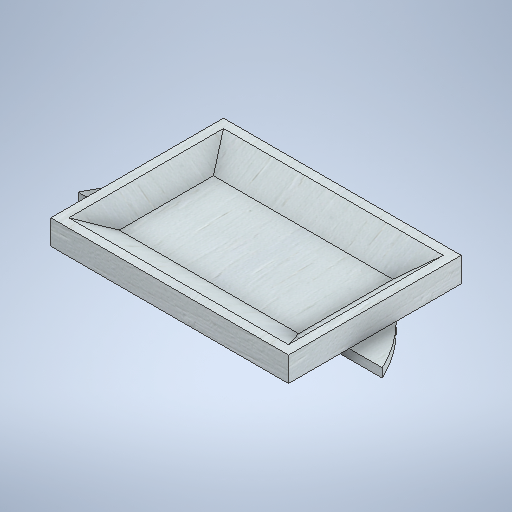
# Autodesk Inventor part: Soporte_caja
Saved by Autodesk Inventor 2025.2 (Build 292293000, 293)
## iProperties
Created: 2025-11-06
Part Number: Soporte_caja
Material: Genérico
Document SubType Name: Modeling
Designer: Dax
Density: 1 g/cm^3
Appearance: Madera - Pintada Blanco
Author: Dax
Autodesk Inventor part; units mm, degrees
ref_plane "YZ Plane" through (0, 0, 0) normal (1, 0, 0) x (0, 1, 0)
ref_plane "XZ Plane" through (0, 0, 0) normal (0, 1, 0) x (-1, 0, 0)
ref_plane "XY Plane" through (0, 0, 0) normal (0, 0, 1) x (1, 0, 0)
sketch "Boceto1" plane through (0, 0, 0) normal (0, 1, 0) x (-1, 0, 0)
  arc A0 (-67.8307, -32) -> (67.8307, -32) centre (0, 0) ccw
  line L0 (0, -32) -> (-67.8307, -32)
  line L1 (0, -32) -> (67.8307, -32)
  dimension "d0" = 150
  constraints: 4 end point, 2 point on circle, 1 centre point, 1 coincident, 1 horizontal
  measures "d0" diameter of A0
extrude "Extrusión1" add sketch "Boceto1" along normal blind 4
sketch "Boceto2" plane through (0, 4, 0) normal (0, 1, 0) x (1, 0, 0)
  line L0 (-67.8307, 32) -> (67.8307, 32) projected
  line L1 (0, 32) -> (0, 5)
  line L2 (0, 5) -> (-53, 5)
  line L3 (-53, 5) -> (-53, 82)
  line L4 (-53, 82) -> (53, 82)
  line L5 (53, 82) -> (53, 5)
  line L6 (53, 5) -> (0, 5)
  point P0 (0, 0)
  dimension "d4" = 27
  dimension "d5" = 53
  dimension "d6" = 77
  dimension "d7" = 106
  constraints: 12 end point, 5 perpendicular, 1 midpoint, 1 point on line, 1 vertical
  measures "d4" distance of L1.start L1.end
  measures "d5" distance of L1.end L2.end
  measures "d6" distance of L2.end L3.end
  measures "d7" distance of L3.end L4.end
extrude "Extrusión2" add sketch "Boceto2" along normal blind 11
sketch "Boceto3" plane through (0, 15, 0) normal (0, 1, 0) x (1, 0, 0)
  line L0 (53, 5) -> (53, 82) projected
  line L1 (53, 43.5) -> (53, 64.5)
  line L2 (40, 64.5) -> (-40, 64.5)
  line L3 (-53, 82) -> (-53, 5) projected
  line L4 (53, 82) -> (-53, 82) projected
  line L5 (0, 82) -> (40, 82)
  line L6 (40, 64.5) -> (40, 22.5)
  line L7 (-53, 5) -> (53, 5) projected
  line L8 (0, 82) -> (-40, 82)
  line L9 (-40, 64.5) -> (-40, 22.5)
  line L10 (53, 43.5) -> (53, 22.5)
  line L11 (40, 22.5) -> (-40, 22.5)
  point P0 (0, 0)
  dimension "d10" = 21
  dimension "d11" = 40
  dimension "d12" = 40
  dimension "d13" = 21
  constraints: 16 end point, 4 point on line, 3 perpendicular, 2 midpoint, 1 horizontal
  measures "d10" distance of L1.start L1.end
  measures "d11" distance of L5.start L5.end
  measures "d12" distance of L5.start L8.end
  measures "d13" distance of L1.start L10.end
extrude "Extrusión3" cut sketch "Boceto3" against normal blind 7 contours L6 L11 L9 L2
sketch "Boceto4" plane through (40, 15, -22.5) normal (0, 0, -1) x (-1, 0, 0)
  line L0 (80, 0) -> (80, -7) projected
  line L1 (0, 0) -> (0, -7) projected
  line L2 (80, -7) -> (0, -7)
  line L3 (-13, 0) -> (-9, 0)
  line L4 (-9, 0) -> (0, 0)
  line L5 (0, 0) -> (0, -7)
  line L6 (0, -7) -> (-9, 0)
  line L7 (93, 0) -> (89, 0)
  line L8 (89, 0) -> (80, 0)
  line L9 (80, -7) -> (89, 0)
  point P0 (40, -15)
  dimension "d16" = 4
  dimension "d17" = 4
  constraints: 16 end point, 3 perpendicular, 2 horizontal
  measures "d16" distance of L3.start L3.end
  measures "d17" distance of L7.start L7.end
extrude "Extrusión4" cut sketch "Boceto4" along normal blind 55.5 and the other way blind 13.5
sketch "Boceto5" plane through (40, 8, -64.5) normal (1, 0, 0) x (0, 0, -1)
  line L0 (0, 7) -> (0, 0) projected
  line L1 (0, 0) -> (0, 7)
  line L2 (13.5, 7) -> (13.5, 0) projected
  line L3 (0, 7) -> (13.5, 7)
  line L4 (0, 0) -> (13.5, 0) projected
  line L5 (13.5, 7) -> (0, 0)
  line L6 (0, 0) -> (0, 7)
  line L7 (-42, 0) -> (0, 0) projected
  line L8 (-42, 7) -> (-42, 0) projected
  line L9 (-42, 0) -> (-42, 7)
  line L10 (-55.5, 7) -> (-55.5, 0) projected
  line L11 (-42, 7) -> (-55.5, 7)
  line L12 (-55.5, 0) -> (-42, 0) projected
  line L13 (-55.5, 7) -> (-42, 0)
  point P0 (-64.5, -8)
  constraints: 14 end point, 3 perpendicular, 2 collinear
extrude "Extrusión5" cut sketch "Boceto5" against normal blind 80 contours L3 L5 L0 | L13 L11 L8
sketch "Boceto6" plane through (40, 8, -78) normal (1, 0, 0) x (0, 0, -1)
  line L0 (-69, 0) -> (-69, 7) projected
  line L1 (-69, 0) -> (-55.5, 0) projected
  line L2 (-69, 7) -> (-69, 0)
  line L3 (-69, 0) -> (-55.5, 0)
  line L4 (-69, 7) -> (0, 7) projected
  line L5 (-55.5, 0) -> (-69, 7)
  line L6 (0, 7) -> (0, 0) projected
  line L7 (0, 7) -> (0, 0)
  line L8 (-13.5, 0) -> (0, 7) projected
  line L9 (0, 0) -> (-13.5, 0)
  line L10 (0, 7) -> (-13.5, 0)
  point P0 (-78, -8)
  constraints: 12 end point, 2 collinear, 1 perpendicular, 1 vertical
extrude "Extrusión6" add sketch "Boceto6" along normal blind 10 and the other way blind 90
